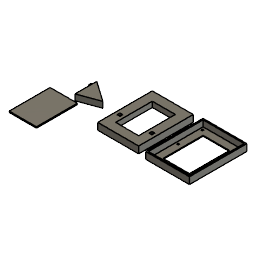
Ramecek (Autodesk Fusion 360 design; units mm, degrees)
Autodesk Fusion 360 part; units mm, degrees
sketch "Sketch1" plane through (0, 0, 0) normal (0, 1, 0) x (1, 0, 0)
  line L0 (75, 100) -> (-75, 100)
  line L1 (-75, 100) -> (-75, -100)
  line L2 (-75, -100) -> (75, -100)
  line L3 (75, -100) -> (75, 100)
  line L4 (75, 100) -> (-75, -100) construction
  line L5 (-75, 100) -> (75, -100) construction
  dimension "d1" = 150
  dimension "d2" = 200
  constraint horizontal L0
  constraint perpendicular L0 L1
  constraint parallel L0 L2
  constraint parallel L1 L3
  constraint coincident L4 origin
  constraint coincident L5 origin
  measures "d1" distance of L1.end L2.end
  measures "d2" distance of L0.end L1.end
extrude "Extrude1" add sketch "Sketch1" along normal blind 25 makes body 1
sketch "Sketch2" plane through (0, 25, 0) normal (0, 1, 0) x (-1, 0, 0)
  line L0 (-75, 100) -> (-75, -100)
  line L1 (-75, -100) -> (75, -100)
  line L2 (75, -100) -> (75, 100)
  line L3 (75, 100) -> (-75, 100)
  line L4 (51, 76) -> (-51, 76)
  line L5 (-51, 76) -> (-51, -76)
  line L6 (-51, -76) -> (51, -76)
  line L7 (51, -76) -> (51, 76)
  line L8 (51, 76) -> (-51, -76) construction
  line L9 (-51, 76) -> (51, -76) construction
  dimension "d5" = 102
  dimension "d6" = 152
  constraint horizontal L4
  constraint perpendicular L4 L5
  constraint parallel L4 L6
  constraint parallel L5 L7
  constraint coincident L8 origin
  constraint coincident L9 origin
  measures "d5" distance of L5.end L6.end
  measures "d6" distance of L4.end L5.end
extrude "Extrude2" cut sketch "Sketch2" against normal blind 5 contours L4 L5 L6 L7 bodies 1
sketch "Sketch3" plane through (0, 20, 0) normal (0, 1, 0) x (-1, 0, 0)
  line L0 (51, -76) -> (51, 76)
  line L1 (51, 76) -> (-51, 76)
  line L2 (-51, 76) -> (-51, -76)
  line L3 (-51, -76) -> (51, -76)
  line L4 (42, 67) -> (-42, 67)
  line L5 (-42, 67) -> (-42, -67)
  line L6 (-42, -67) -> (42, -67)
  line L7 (42, -67) -> (42, 67)
  line L8 (42, 67) -> (-42, -67) construction
  line L9 (-42, 67) -> (42, -67) construction
  dimension "d9" = 84
  dimension "d10" = 134
  constraint horizontal L4
  constraint perpendicular L4 L5
  constraint parallel L4 L6
  constraint parallel L5 L7
  constraint coincident L8 origin
  constraint coincident L9 origin
  measures "d9" distance of L5.end L6.end
  measures "d10" distance of L4.end L5.end
extrude "Extrude3" cut sketch "Sketch3" against normal blind 20 contours L4 L5 L6 L7 bodies 1
sketch "Sketch4" plane through (0, 0, 0) normal (0, 1, 0) x (1, 0, 0)
  line L0 (275.15, 100.05) -> (124.95, 100.05)
  line L1 (124.95, 100.05) -> (124.95, -100.15)
  line L2 (124.95, -100.15) -> (275.15, -100.15)
  line L3 (275.15, -100.15) -> (275.15, 100.05)
  line L4 (275.15, 100.05) -> (124.95, -100.15) construction
  line L5 (124.95, 100.05) -> (275.15, -100.15) construction
  line L6 (119.95, 105.05) -> (119.95, -105.15)
  line L7 (119.95, -105.15) -> (280.15, -105.15)
  line L8 (280.15, -105.15) -> (280.15, 105.05)
  line L9 (280.15, 105.05) -> (119.95, 105.05)
  line L10 (152.05, -73.05) -> (248.05, -73.05)
  line L11 (248.05, -73.05) -> (248.05, 72.95)
  line L12 (248.05, 72.95) -> (152.05, 72.95)
  line L13 (152.05, 72.95) -> (152.05, -73.05)
  line L14 (152.05, -73.05) -> (248.05, 72.95) construction
  line L15 (248.05, -73.05) -> (152.05, 72.95) construction
  point P0 (200.05, -0.05)
  point P1 (200.05, -0.05)
  dimension "d13" = 150.2
  dimension "d14" = 200.2
  dimension "d15" = 5
  dimension "d22" = 96
  dimension "d23" = 146
  constraint horizontal L0
  constraint perpendicular L0 L1
  constraint parallel L0 L2
  constraint parallel L1 L3
  constraint coincident L4 P1
  constraint coincident L5 P1
  constraint horizontal L10
  constraint perpendicular L10 L11
  constraint parallel L10 L12
  constraint parallel L11 L13
  constraint coincident L14 P1
  constraint coincident L15 P1
  constraint coincident P1 P0
  measures "d13" distance of L1.end L2.end
  measures "d14" distance of L0.end L1.end
  measures "d22" distance of L11.end L12.end
  measures "d23" distance of L10.end L11.end
extrude "Extrude4" add sketch "Sketch4" along normal blind 25 separate body contours L6 L7 L8 L9 makes body 2
extrude "Extrude5" add sketch "Sketch4" along normal blind 3 contours L0 L1 L2 L3 | L10 L11 L12 L13 bodies 2
extrude "Extrude6" cut sketch "Sketch4" along normal blind 10 contours L10 L11 L12 L13 bodies 2
move_body "Move1" bodies 2 to x (1, 0, 0) y (0, -1, 0) z (0, 0, -1) at (0, 50, 210.3)
move_body "Move2" bodies 2 to x (1, 0, 0) y (0, 1, 0) z (0, 0, 1) at (0, 0, -210)
sketch "Sketch6" plane through (0, 50, 0) normal (0, 1, 0) x (-1, 0, 0)
  line L0 (-248.05, 73.25) -> (-152.05, 73.25)
  line L1 (-152.05, 73.25) -> (-152.05, -72.75)
  line L2 (-152.05, -72.75) -> (-248.05, -72.75)
  line L3 (-248.05, -72.75) -> (-248.05, 73.25)
  line L4 (-119.95, 105.35) -> (-280.15, 105.35)
  line L5 (-280.15, 105.35) -> (-280.15, -104.85)
  line L6 (-280.15, -104.85) -> (-119.95, -104.85)
  line L7 (-119.95, -104.85) -> (-119.95, 105.35)
  line L8 (-263.85, 86.7) -> (-269.05, 86.7)
  line L9 (-269.05, 86.7) -> (-269.05, 91.9)
  line L10 (-269.05, 91.9) -> (-263.85, 91.9)
  line L11 (-263.85, 91.9) -> (-263.85, 86.7)
  line L12 (-263.85, 86.7) -> (-269.05, 91.9) construction
  line L13 (-269.05, 86.7) -> (-263.85, 91.9) construction
  line L14 (-395.5406, 0.25) -> (-164.7594, 0.25)
  line L15 (-200.05, 237.6573) -> (-200.05, -26.9573)
  line L16 (-131.05, 91.9) -> (-136.25, 91.9)
  line L17 (-131.05, 86.7) -> (-131.05, 91.9)
  line L18 (-136.25, 86.7) -> (-131.05, 86.7)
  line L19 (-136.25, 91.9) -> (-136.25, 86.7)
  line L20 (-136.25, -91.4) -> (-136.25, -86.2)
  line L21 (-131.05, -91.4) -> (-136.25, -91.4)
  line L22 (-136.25, -86.2) -> (-131.05, -86.2)
  line L23 (-131.05, -86.2) -> (-131.05, -91.4)
  line L24 (-263.85, -86.2) -> (-269.05, -86.2)
  line L25 (-269.05, -86.2) -> (-269.05, -91.4)
  line L26 (-269.05, -91.4) -> (-263.85, -91.4)
  line L27 (-263.85, -91.4) -> (-263.85, -86.2)
  line L28 (-263.85, 2.85) -> (-263.85, -2.35)
  line L29 (-269.05, 2.85) -> (-263.85, 2.85)
  line L30 (-269.05, -2.35) -> (-269.05, 2.85)
  line L31 (-263.85, -2.35) -> (-269.05, -2.35)
  line L32 (-131.05, 2.85) -> (-136.25, 2.85)
  line L33 (-131.05, -2.35) -> (-131.05, 2.85)
  line L34 (-136.25, -2.35) -> (-131.05, -2.35)
  line L35 (-136.25, 2.85) -> (-136.25, -2.35)
  point P0 (-266.45, 89.3)
  point P1 (-266.45, 89.3)
  dimension "d27" = 5.2
  dimension "d28" = 5.2
  dimension "d36" = 5.2
  dimension "d37" = 5.2
  dimension "d38" = 2.6
  dimension "d117" = 11.1
  dimension "d118" = 11.1
  constraint horizontal L8
  constraint perpendicular L8 L9
  constraint parallel L8 L10
  constraint parallel L9 L11
  constraint coincident L12 P1
  constraint coincident L13 P1
  constraint coincident P1 P0
  constraint perpendicular L7 L14
  constraint midpoint L5 L14
  constraint perpendicular L6 L15
  constraint midpoint L4 L15
  constraint symmetric L8.start L15 L18.start
  constraint symmetric L8.end L15 L17.start
  constraint symmetric L9.end L15 L16.start
  constraint symmetric L10.end L15 L16.end
  constraint symmetric L8.start L14 L24.start
  constraint symmetric L8.end L14 L24.end
  constraint symmetric L9.end L14 L25.end
  constraint symmetric L10.end L14 L26.end
  constraint symmetric L14 L16.start L21.start
  constraint symmetric L14 L16.end L20.start
  constraint symmetric L14 L17.start L22.end
  constraint symmetric L14 L18.start L20.end
  constraint horizontal L31
  constraint perpendicular L30 L31
  constraint parallel L29 L31
  constraint parallel L28 L30
  constraint symmetric L15 L28.start L32.end
  constraint symmetric L15 L29.start L32.start
  constraint symmetric L15 L28.end L34.start
  constraint symmetric L15 L30.start L33.start
  measures "d27" distance of L9.end L10.end
  measures "d28" distance of L8.end L9.end
  measures "d36" distance of L28.start L29.start
  measures "d37" distance of L29.start L30.start
  measures "d38" distance of L14 L28.start
  measures "d117" distance of L5 L9
  measures "d118" distance of L5 L30
move_body "Move3" bodies 1 to x (1, 0, 0) y (0, -1, 0) z (0, 0, -1) at (0, 50, -200)
move_body "Move4" bodies 1 to x (1, 0, 0) y (0, 1, 0) z (0, 0, 1) at (0, 0, 210)
extrude "Extrude8" cut sketch "Sketch6" against normal blind 100 contours L14 L28 L30 L31 | L14 L28 L29 L30 | L8 L9 L10 L11 | L16 L17 L18 L19 | L20 L21 L22 L23 | L24 L25 L26 L27 | L32 L33 L34 L35 bodies 2
move_body "Move5" bodies 1 to x (-1, 0, 0) y (0, -1, 0) z (0, 0, 1) at (-150, 100, 0)
move_body "Move6" bodies 1 to x (1, 0, 0) y (0, 1, 0) z (0, 0, 1) at (169.7139, 0, -8.0413)
move_body "Move7" bodies 2 to x (-1, 0, 0) y (0, -1, 0) z (0, 0, 1) at (239.9, 100, 0)
move_body "Move8" bodies 2 to x (1, 0, 0) y (0, 1, 0) z (0, 0, 1) at (155.1893, 0, 0.7244)
sketch "Sketch10" plane through (0, 75, 0) normal (0, 1, 0) x (-1, 0, 0)
  line L0 (31.2861, -74.0413) -> (-70.7139, -74.0413)
  line L1 (-70.7139, -74.0413) -> (-70.7139, 77.9587)
  line L2 (-70.7139, 77.9587) -> (31.2861, 77.9587)
  line L3 (31.2861, 77.9587) -> (31.2861, -74.0413)
  line L4 (55.2861, -98.0413) -> (55.2861, 101.9587)
  line L5 (55.2861, 101.9587) -> (-94.7139, 101.9587)
  line L6 (-94.7139, 101.9587) -> (-94.7139, -98.0413)
  line L7 (-94.7139, -98.0413) -> (55.2861, -98.0413)
  line L8 (-19.7139, 163.9174) -> (-19.7139, 40)
  line L9 (-153.633, 1.9587) -> (-35.7948, 1.9587)
  line L10 (-88.7139, 88.3087) -> (-83.5139, 88.3087)
  line L11 (-83.5139, 88.3087) -> (-83.5139, 93.5087)
  line L12 (-83.5139, 93.5087) -> (-88.7139, 93.5087)
  line L13 (-88.7139, 93.5087) -> (-88.7139, 88.3087)
  line L14 (-88.7139, 88.3087) -> (-83.5139, 93.5087) construction
  line L15 (-83.5139, 88.3087) -> (-88.7139, 93.5087) construction
  line L16 (44.0861, 93.5087) -> (49.2861, 93.5087)
  line L17 (49.2861, 93.5087) -> (49.2861, 88.3087)
  line L18 (49.2861, 88.3087) -> (44.0861, 88.3087)
  line L19 (44.0861, 88.3087) -> (44.0861, 93.5087)
  line L20 (-88.7139, -89.5913) -> (-88.7139, -84.3913)
  line L21 (-83.5139, -89.5913) -> (-88.7139, -89.5913)
  line L22 (-83.5139, -84.3913) -> (-83.5139, -89.5913)
  line L23 (-88.7139, -84.3913) -> (-83.5139, -84.3913)
  line L24 (44.0861, -84.3913) -> (44.0861, -89.5913)
  line L25 (49.2861, -84.3913) -> (44.0861, -84.3913)
  line L26 (49.2861, -89.5913) -> (49.2861, -84.3913)
  line L27 (44.0861, -89.5913) -> (49.2861, -89.5913)
  line L28 (-88.7139, 4.5587) -> (-88.7139, -0.6413)
  line L29 (-88.7139, -0.6413) -> (-83.5139, -0.6413)
  line L30 (-83.5139, -0.6413) -> (-83.5139, 4.5587)
  line L31 (-83.5139, 4.5587) -> (-88.7139, 4.5587)
  line L32 (44.0861, 4.5587) -> (49.2861, 4.5587)
  line L33 (49.2861, 4.5587) -> (49.2861, -0.6413)
  line L34 (49.2861, -0.6413) -> (44.0861, -0.6413)
  line L35 (44.0861, -0.6413) -> (44.0861, 4.5587)
  point P0 (-86.1139, 90.9087)
  dimension "d112" = 5.2
  dimension "d113" = 5.2
  dimension "d114" = 5.2
  dimension "d115" = 5.2
  dimension "d119" = 6
  dimension "d120" = 8.45
  dimension "d121" = 6
  constraint vertical L8
  constraint midpoint L5 L8
  constraint perpendicular L1 L9
  constraint midpoint L6 L9
  constraint horizontal L10
  constraint perpendicular L10 L11
  constraint parallel L10 L12
  constraint parallel L11 L13
  constraint coincident L14 P0
  constraint coincident L15 P0
  constraint symmetric L8 L10.start L17.end
  constraint symmetric L8 L10.end L18.end
  constraint symmetric L8 L11.end L16.start
  constraint symmetric L8 L12.end L16.end
  constraint symmetric L9 L10.start L20.end
  constraint symmetric L9 L10.end L22.start
  constraint symmetric L9 L11.end L21.start
  constraint symmetric L9 L12.end L20.start
  constraint symmetric L9 L16.start L24.end
  constraint symmetric L9 L16.end L26.start
  constraint symmetric L9 L17.end L25.start
  constraint symmetric L9 L18.end L24.start
  constraint horizontal L29
  constraint perpendicular L29 L30
  constraint parallel L29 L31
  constraint parallel L28 L30
  constraint symmetric L8 L28.end L33.end
  constraint symmetric L8 L29.end L34.end
  constraint symmetric L8 L30.end L32.start
  constraint symmetric L8 L28.start L32.end
  measures "d112" distance of L11.end L12.end
  measures "d113" distance of L10.end L11.end
  measures "d114" distance of L30.end L28.start
  measures "d115" distance of L29.end L30.end
  measures "d119" distance of L6 L13
  measures "d120" distance of L5 L12
  measures "d121" distance of L6 L28
extrude "Extrude12" cut sketch "Sketch10" against normal blind 3.5 contours L9 L28 L29 L30 | L9 L28 L30 L31 | L10 L11 L12 L13 | L16 L17 L18 L19 | L20 L21 L22 L23 | L24 L25 L26 L27 | L32 L33 L34 L35 bodies 1
move_body "Move9" bodies 1 to x (-1, 0, 0) y (0, -1, 0) z (0, 0, 1) at (-110.5722, 150, 0)
move_body "Move10" bodies 1 to x (1, 0, 0) y (0, 1, 0) z (0, 0, 1) at (140.3925, -24.7351, 0)
sketch "Sketch11" plane through (0, 0, 0) normal (0, 1, 0) x (1, 0, 0)
  line L0 (-250, 0) -> (-250, 80)
  line L1 (-320, 0) -> (-80, 0)
  line L2 (-250, 0) -> (-174.8246, 27.3616)
  line L3 (-250, 0) -> (-190, 0) construction
  line L4 (-250, 80) -> (-174.8246, 27.3616)
  dimension "d83" = 80
  dimension "d84" = 80
  dimension "d85" = 20
  constraint vertical L0
  constraint perpendicular L0 L1
  constraint horizontal L3
  measures "d83" distance of L0.start L0.end
  measures "d84" distance of L0.start L2.end
  measures "d85" angle of L2 L3
extrude "Extrude13" add sketch "Sketch11" along normal blind 22 separate body makes body 3
sketch "Sketch12" plane through (-250, 0, 0) normal (-1, 0, 0) x (0, 0, 1)
  line L0 (-80, 0) -> (0, 0)
  line L1 (0, 0) -> (0, 22)
  line L2 (0, 22) -> (-80, 22)
  line L3 (-80, 22) -> (-80, 0)
  line L4 (-132.5, 11) -> (-27.5, 11)
  line L5 (-60, 16) -> (-70, 16)
  line L6 (-70, 16) -> (-70, 6)
  line L7 (-70, 6) -> (-60, 6)
  line L8 (-60, 6) -> (-60, 16)
  line L9 (-60, 16) -> (-70, 6) construction
  line L10 (-70, 16) -> (-60, 6) construction
  point P0 (-65, 11)
  dimension "d88" = 10
  dimension "d91" = 10
  dimension "d94" = 10
  constraint horizontal L4
  constraint midpoint L3 L4
  constraint horizontal L5
  constraint perpendicular L5 L6
  constraint parallel L5 L7
  constraint parallel L6 L8
  constraint coincident L9 P0
  constraint coincident L10 P0
  constraint coincident L4 P0
  measures "d88" distance of L3 L6
  measures "d91" distance of L5 L7
  measures "d94" distance of L6 L8
extrude "Extrude14" add sketch "Sketch12" along normal blind 10 contours L4 L5 L6 L8 | L4 L6 L7 L8 bodies 3
sketch "Sketch16" plane through (0, 50.2649, 0) normal (0, -1, 0) x (1, 0, 0)
  line L0 (-63.5651, 41) -> (-41.0651, 41)
  line L1 (-41.0651, 41) -> (-41.0651, 19)
  line L2 (-41.0651, 19) -> (-63.5651, 19)
  line L3 (-63.5651, 19) -> (-63.5651, 41)
  line L4 (-63.5651, 41) -> (-41.0651, 19) construction
  line L5 (-41.0651, 41) -> (-63.5651, 19) construction
  line L6 (-58.8936, 4.5587) -> (-53.6936, 4.5587)
  line L7 (-58.8936, -0.6413) -> (-58.8936, 4.5587)
  line L8 (-53.6936, -0.6413) -> (-58.8936, -0.6413)
  line L9 (-53.6936, 4.5587) -> (-53.6936, -0.6413)
  line L10 (79.1064, 93.5087) -> (79.1064, 88.3087)
  line L11 (79.1064, 88.3087) -> (73.9064, 88.3087)
  line L12 (73.9064, 88.3087) -> (73.9064, 93.5087)
  line L13 (73.9064, 93.5087) -> (79.1064, 93.5087)
  line L14 (79.1064, -84.3913) -> (79.1064, -89.5913)
  line L15 (79.1064, -89.5913) -> (73.9064, -89.5913)
  line L16 (73.9064, -89.5913) -> (73.9064, -84.3913)
  line L17 (73.9064, -84.3913) -> (79.1064, -84.3913)
  line L18 (-53.6936, 88.3087) -> (-58.8936, 88.3087)
  line L19 (-58.8936, 88.3087) -> (-58.8936, 93.5087)
  line L20 (-58.8936, 93.5087) -> (-53.6936, 93.5087)
  line L21 (-53.6936, 93.5087) -> (-53.6936, 88.3087)
  line L22 (79.1064, 4.5587) -> (79.1064, -0.6413)
  line L23 (79.1064, -0.6413) -> (73.9064, -0.6413)
  line L24 (73.9064, -0.6413) -> (73.9064, 4.5587)
  line L25 (73.9064, 4.5587) -> (79.1064, 4.5587)
  line L26 (-53.6936, -89.5913) -> (-58.8936, -89.5913)
  line L27 (-58.8936, -89.5913) -> (-58.8936, -84.3913)
  line L28 (-58.8936, -84.3913) -> (-53.6936, -84.3913)
  line L29 (-53.6936, -84.3913) -> (-53.6936, -89.5913)
  line L30 (61.1064, -74.0413) -> (-40.8936, -74.0413)
  line L31 (-40.8936, -74.0413) -> (-40.8936, 77.9587)
  line L32 (-40.8936, 77.9587) -> (61.1064, 77.9587)
  line L33 (61.1064, 77.9587) -> (61.1064, -74.0413)
  line L34 (85.1064, -98.0413) -> (85.1064, 101.9587)
  line L35 (85.1064, 101.9587) -> (-64.8936, 101.9587)
  line L36 (-64.8936, 101.9587) -> (-64.8936, -98.0413)
  line L37 (-64.8936, -98.0413) -> (85.1064, -98.0413)
  point P0 (-52.3151, 30)
  dimension "d110" = 22.5
  dimension "d111" = 22
  constraint horizontal L0
  constraint perpendicular L0 L1
  constraint parallel L0 L2
  constraint parallel L1 L3
  constraint coincident L4 P0
  constraint coincident L5 P0
  measures "d110" distance of L1.end L2.end
  measures "d111" distance of L0.end L1.end
sketch "Sketch17" plane through (0, 75.2649, 0) normal (0, 1, 0) x (-1, 0, 0)
  line L0 (31.8936, -65.0413) -> (-52.1064, -65.0413)
  line L1 (-52.1064, -65.0413) -> (-52.1064, 68.9587)
  line L2 (-52.1064, 68.9587) -> (31.8936, 68.9587)
  line L3 (31.8936, 68.9587) -> (31.8936, -65.0413)
  line L4 (-85.1064, 101.9587) -> (-85.1064, -98.0413)
  line L5 (-85.1064, -98.0413) -> (64.8936, -98.0413)
  line L6 (64.8936, -98.0413) -> (64.8936, 101.9587)
  line L7 (64.8936, 101.9587) -> (-85.1064, 101.9587)
  line L8 (53.4936, 41.9587) -> (43.2936, 41.9587)
  line L9 (43.2936, 41.9587) -> (43.2936, 31.7587)
  line L10 (43.2936, 31.7587) -> (53.4936, 31.7587)
  line L11 (53.4936, 31.7587) -> (53.4936, 41.9587)
  line L12 (53.4936, 41.9587) -> (43.2936, 31.7587) construction
  line L13 (43.2936, 41.9587) -> (53.4936, 31.7587) construction
  line L14 (-10.1064, -84.9903) -> (-10.1064, -45.0923)
  line L15 (-63.5064, 41.9587) -> (-63.5064, 31.7587)
  line L16 (-63.5064, 31.7587) -> (-73.7064, 31.7587)
  line L17 (-73.7064, 31.7587) -> (-73.7064, 41.9587)
  line L18 (-73.7064, 41.9587) -> (-63.5064, 41.9587)
  point P0 (48.3936, 36.8587)
  dimension "d122" = 10.2
  dimension "d123" = 10.2
  dimension "d124" = 60
  dimension "d125" = 16.5
  constraint horizontal L8
  constraint perpendicular L8 L9
  constraint parallel L8 L10
  constraint parallel L9 L11
  constraint coincident L12 P0
  constraint coincident L13 P0
  constraint vertical L14
  constraint midpoint L0 L14
  constraint symmetric L8.start L14 L17.end
  constraint symmetric L8.end L14 L15.start
  constraint symmetric L9.end L14 L15.end
  constraint symmetric L10.end L14 L16.end
  measures "d122" distance of L9.end L10.end
  measures "d123" distance of L8.end L9.end
  measures "d124" distance of L7 L8
  measures "d125" distance of L3 P0
extrude "Extrude18" cut sketch "Sketch17" against normal blind 10.2 contours L8 L9 L10 L11 | L15 L16 L17 L18 bodies 1
sketch "Sketch18" plane through (0, 0, 0) normal (0, 1, 0) x (1, 0, 0)
  line L0 (-233.4125, -7.3986) -> (-333.4125, -7.3986)
  line L1 (-333.4125, -7.3986) -> (-333.4125, -157.3986)
  line L2 (-333.4125, -157.3986) -> (-233.4125, -157.3986)
  line L3 (-233.4125, -157.3986) -> (-233.4125, -7.3986)
  line L4 (-233.4125, -7.3986) -> (-333.4125, -157.3986) construction
  line L5 (-333.4125, -7.3986) -> (-233.4125, -157.3986) construction
  point P0 (-283.4125, -82.3986)
  dimension "d128" = 100
  dimension "d129" = 150
  constraint horizontal L0
  constraint perpendicular L0 L1
  constraint parallel L0 L2
  constraint parallel L1 L3
  constraint coincident L4 P0
  constraint coincident L5 P0
  measures "d128" distance of L1.end L2.end
  measures "d129" distance of L0.end L1.end
extrude "Extrude19" add sketch "Sketch18" along normal blind 4.5 separate body makes body 4
equation "d1 = 10 cm + 5 cm"
equation "d2 = 15 cm + 5 cm"
equation "d9 = 10 cm - 1.6 cm"
equation "d10 = 15 cm - 1.6 cm"
equation "d22 = 100 mm - 4 mm"
equation "d23 = 150 mm - 4 mm"
equation "d38 = ( 5.2 / 2 ) * 1 mm"
equation "d117 = 5.1 mm + 6 mm"
equation "d118 = 5.1 mm + 6 mm"
equation "d125 = ( 33 / 2 ) * 1 mm"
